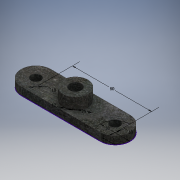
# Autodesk Inventor part: Крышка
Saved by Autodesk Inventor 2018 (Build 220112000, 112)
## iProperties
Created: 2020-04-13
Part Number: Крышка
Material: Сталь
Document SubType Name: ЛистМат
Designer: Alena Oparina
Density: 7.85 g/cm^3
Appearance: Листовая
Sheet Metal Rule: По умолчанию_мм
Author: Alena Oparina
Autodesk Inventor part; units mm, degrees
ref_plane "YZ Plane" through (0, 0, 0) normal (1, 0, 0) x (0, 1, 0)
ref_plane "XZ Plane" through (0, 0, 0) normal (0, 1, 0) x (-1, 0, 0)
ref_plane "XY Plane" through (0, 0, 0) normal (0, 0, 1) x (1, 0, 0)
sketch "Эскиз1" plane through (0, 0, 0) normal (0, 0, 1) x (1, 0, 0)
  line L0 (0, 0) -> (80, 0) construction
  line L1 (0, -15) -> (80, -15)
  line L2 (80, 15) -> (0, 15)
  arc A0 (0, 15) -> (0, -15) centre (0, 0) ccw
  arc A1 (80, -15) -> (80, 15) centre (80, 0) ccw
  circle A2 centre (40, 0) radius 12.5
  circle A3 centre (80, 0) radius 5
  circle A4 centre (0, 0) radius 5
  circle A5 centre (40, 0) radius 6
  dimension "d0" = 80
  dimension "d1" = 30
  dimension "d4" = 25
  dimension "d5" = 10
  dimension "d6" = 10
  dimension "d7" = 12
  constraints: 8 end point, 6 centre point, 4 coincident, 4 point on circle, 4 tangent, 1 horizontal, 1 midpoint, 1 parallel
  measures "d0" distance of L0.start L0.end
  measures "d1" diameter of A1
  measures "d4" diameter of A2
  measures "d5" diameter of A3
  measures "d6" diameter of A4
  measures "d7" diameter of A5
extrude "Выдавливание1" add sketch "Эскиз1" along normal blind 8 contours A0 L2 A1 L1 | A2 | A3 | A4 | A5
extrude "Выдавливание2" cut sketch "Эскиз1" along normal up to next contours A5
extrude "Выдавливание3" add sketch "Эскиз1" along normal blind 20 contours A2
extrude "Выдавливание4" cut sketch "Эскиз1" along normal up to next contours A3 | A4
equation "\"Радиус_гибки\" = Толщина"
equation "\"Ширина_просечки\" = Толщина"
equation "\"Глубина_просечки\" = 0.5 * Толщина"
equation "\"Размер_просечки\" = 4 * Толщина"
equation "\"Мин_остаток\" = 2 * Толщина"
equation "\"Радиус_перехода\" = Радиус_гибки"
equation "\"Радиус_Якоби\" = Радиус_гибки"
equation "\"Размер_зазора\" = Толщина"
equation "\"Толщина\" = 8"
